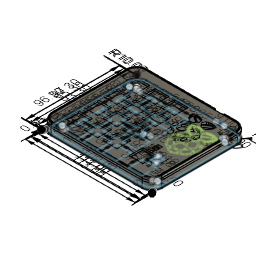
Raspberry pi pico Macropad (Autodesk Fusion 360 design; units mm, degrees)
Autodesk Fusion 360 part; units mm, degrees
sketch "Sketch1" plane through (0, 0, 0) normal (0, 0, 1) x (1, 0, 0)
  line L0 (12, 3) -> (101, 3)
  line L1 (111, 13) -> (111, 86.3)
  line L2 (101, 96.3) -> (12, 96.3)
  line L3 (2, 86.3) -> (2, 13)
  line L4 (11, 1) -> (102, 1)
  line L5 (112, 11) -> (112, 86.3)
  line L6 (102, 96.3) -> (11, 96.3)
  line L7 (1, 86.3) -> (1, 11)
  line L8 (10, 0) -> (103, 0)
  line L9 (113, 10) -> (113, 87.3)
  line L10 (103, 97.3) -> (10, 97.3)
  line L11 (0, 87.3) -> (0, 10)
  arc A0 (12, 96.3) -> (2, 86.3) centre (12, 86.3) ccw
  arc A1 (11, 96.3) -> (1, 86.3) centre (11, 86.3) ccw
  arc A2 (10, 97.3) -> (0, 87.3) centre (10, 87.3) ccw
  arc A3 (111, 86.3) -> (101, 96.3) centre (101, 86.3) ccw
  arc A4 (112, 86.3) -> (102, 96.3) centre (102, 86.3) ccw
  arc A5 (113, 87.3) -> (103, 97.3) centre (103, 87.3) ccw
  arc A6 (101, 3) -> (111, 13) centre (101, 13) ccw
  arc A7 (102, 1) -> (112, 11) centre (102, 11) ccw
  arc A8 (103, 0) -> (113, 10) centre (103, 10) ccw
  arc A9 (2, 13) -> (12, 3) centre (12, 13) ccw
  arc A10 (1, 11) -> (11, 1) centre (11, 11) ccw
  arc A11 (0, 10) -> (10, 0) centre (10, 10) ccw
  circle A12 centre (7, 82.9) radius 2.5
  circle A13 centre (105, 82.5) radius 2.5
  circle A14 centre (105, 13.8) radius 2.5
  circle A15 centre (7, 14.2) radius 2.5
  line L12 (56, 48.35) -> (56, 50.35)
  line L13 (56, 50.35) -> (53.5, 46.0199)
  line L14 (56, 50.35) -> (61, 50.35) construction
  line L15 (56, 50.35) -> (58.5, 46.0199)
  line L16 (58.5, 46.0199) -> (53.5, 46.0199)
  circle A16 centre (105, 13.8) radius 1.25
  circle A17 centre (105, 82.5) radius 1.25
  circle A18 centre (7, 82.9) radius 1.25
  circle A19 centre (7, 14.2) radius 1.25
  line L17 (0, 0) -> (0, 0.5)
  line L18 (0, 0.5) -> (0.5, 0.5)
  line L19 (10.5, 0.5) -> (102.5, 0.5)
  line L20 (112.5, 10.5) -> (112.5, 86.8)
  line L21 (102.5, 96.8) -> (10.5, 96.8)
  line L22 (0.5, 86.8) -> (0.5, 10.5)
  arc A20 (112.5, 86.8) -> (102.5, 96.8) centre (102.5, 86.8) ccw
  arc A21 (10.5, 96.8) -> (0.5, 86.8) centre (10.5, 86.8) ccw
  arc A22 (0.5, 10.5) -> (10.5, 0.5) centre (10.5, 10.5) ccw
  arc A23 (102.5, 0.5) -> (112.5, 10.5) centre (102.5, 10.5) ccw
  line L23 (90, 96.3) -> (81, 96.3)
  line L24 (81, 97.3) -> (90, 97.3)
  line L25 (81, 96.3) -> (90, 96.3)
  line L26 (91, 96.3) -> (82, 96.3)
  line L27 (91, 96.3) -> (82, 96.3)
  line L28 (82, 96.3) -> (82, 97.3)
  line L29 (82, 97.3) -> (91, 97.3)
  line L30 (91, 97.3) -> (91, 96.3)
  line L31 (90, 96.3) -> (81, 96.3)
  line L32 (81, 96.3) -> (81, 97.3)
  line L33 (81, 97.3) -> (90, 97.3)
  line L34 (90, 97.3) -> (90, 96.3)
  line L35 (16.9465, 83.797) -> (12.922, 83.797)
  line L36 (12.922, 83.797) -> (12.922, 84.0729)
  line L37 (12.922, 83.797) -> (26.9174, 83.797)
  line L38 (26.9174, 83.797) -> (26.9174, 69.8016)
  line L39 (26.9174, 69.8016) -> (12.922, 69.8016)
  line L40 (12.922, 69.8016) -> (12.922, 83.797)
  line L41 (26.9174, 83.797) -> (32.5054, 83.797)
  line L42 (32.5054, 83.797) -> (46.5008, 83.797)
  line L43 (46.5008, 83.797) -> (46.5008, 69.8016)
  line L44 (46.5008, 69.8016) -> (32.5054, 69.8016)
  line L45 (32.5054, 69.8016) -> (32.5054, 83.797)
  line L46 (46.5008, 83.797) -> (52.0888, 83.797)
  line L47 (52.0888, 83.797) -> (66.0842, 83.797)
  line L48 (66.0842, 83.797) -> (66.0842, 69.8016)
  line L49 (66.0842, 69.8016) -> (52.0888, 69.8016)
  line L50 (52.0888, 69.8016) -> (52.0888, 83.797)
  line L51 (12.922, 69.8016) -> (12.922, 64.2136)
  line L52 (12.922, 64.2136) -> (26.9174, 64.2136)
  line L53 (26.9174, 64.2136) -> (26.9174, 50.2182)
  line L54 (26.9174, 50.2182) -> (12.922, 50.2182)
  line L55 (12.922, 50.2182) -> (12.922, 64.2136)
  line L56 (26.9174, 64.2136) -> (32.5054, 64.2136)
  line L57 (32.5054, 64.2136) -> (46.5008, 64.2136)
  line L58 (46.5008, 64.2136) -> (46.5008, 50.2182)
  line L59 (46.5008, 50.2182) -> (32.5054, 50.2182)
  line L60 (32.5054, 50.2182) -> (32.5054, 64.2136)
  line L61 (46.5008, 64.2136) -> (52.0888, 64.2136)
  line L62 (52.0888, 64.2136) -> (66.0842, 64.2136)
  line L63 (66.0842, 64.2136) -> (66.0842, 50.2182)
  line L64 (66.0842, 50.2182) -> (52.0888, 50.2182)
  line L65 (52.0888, 50.2182) -> (52.0888, 64.2136)
  line L66 (12.922, 50.2182) -> (12.922, 44.6302)
  line L67 (12.922, 44.6302) -> (26.9174, 44.6302)
  line L68 (26.9174, 44.6302) -> (26.9174, 30.6348)
  line L69 (26.9174, 30.6348) -> (12.922, 30.6348)
  line L70 (12.922, 30.6348) -> (12.922, 44.6302)
  line L71 (32.5054, 44.6302) -> (46.5008, 44.6302)
  line L72 (46.5008, 44.6302) -> (46.5008, 30.6348)
  line L73 (46.5008, 30.6348) -> (32.5054, 30.6348)
  line L74 (32.5054, 30.6348) -> (32.5054, 44.6302)
  line L75 (52.0888, 44.6302) -> (66.0842, 44.6302)
  line L76 (66.0842, 44.6302) -> (66.0842, 30.6348)
  line L77 (66.0842, 30.6348) -> (52.0888, 30.6348)
  line L78 (52.0888, 30.6348) -> (52.0888, 44.6302)
  line L79 (12.922, 30.6348) -> (12.922, 25.0468)
  line L80 (12.922, 25.0468) -> (26.9174, 25.0468)
  line L81 (26.9174, 25.0468) -> (26.9174, 11.0514)
  line L82 (26.9174, 11.0514) -> (12.922, 11.0514)
  line L83 (12.922, 11.0514) -> (12.922, 25.0468)
  line L84 (32.5054, 25.0468) -> (46.5008, 25.0468)
  line L85 (46.5008, 25.0468) -> (46.5008, 11.0514)
  line L86 (46.5008, 11.0514) -> (32.5054, 11.0514)
  line L87 (32.5054, 11.0514) -> (32.5054, 25.0468)
  line L88 (52.0888, 25.0468) -> (66.0842, 25.0468)
  line L89 (66.0842, 25.0468) -> (66.0842, 11.0514)
  line L90 (66.0842, 11.0514) -> (52.0888, 11.0514)
  line L91 (52.0888, 11.0514) -> (52.0888, 25.0468)
  line L92 (78.4702, 25.0468) -> (92.4656, 25.0468)
  line L93 (92.4656, 25.0468) -> (92.4656, 11.0514)
  line L94 (92.4656, 11.0514) -> (78.4702, 11.0514)
  line L95 (78.4702, 11.0514) -> (78.4702, 25.0468)
  line L96 (83.3562, 29.7458) -> (87.6742, 29.7458)
  line L97 (87.6742, 29.7458) -> (87.6742, 32.2858)
  line L98 (87.6742, 32.2858) -> (83.3562, 32.2858)
  line L99 (83.3562, 32.2858) -> (83.3562, 29.7458)
  line L100 (83.3562, 32.2858) -> (83.3562, 33.3018)
  line L101 (83.3562, 33.3018) -> (87.6742, 33.3018)
  line L102 (87.6742, 33.3018) -> (87.6742, 35.8418)
  line L103 (87.6742, 35.8418) -> (83.3562, 35.8418)
  line L104 (83.3562, 35.8418) -> (83.3562, 33.3018)
  spline S0 degree 3 poles (79.019, 82.9251) (78.832, 82.9193) (78.6306, 82.8502) (78.4021, 82.67) knots 0 0 0 0 1 1 1 1
  spline S1 degree 3 poles (78.4021, 82.67) (77.8427, 82.8857) (77.2999, 82.9607) (76.8147, 82.5215) knots 0 0 0 0 1 1 1 1
  spline S2 degree 3 poles (76.8147, 82.5215) (76.0654, 82.6186) (75.822, 82.4181) (75.6375, 82.1839) knots 0 0 0 0 1 1 1 1
  spline S3 degree 3 poles (75.6375, 82.1839) (75.473, 82.1873) (74.4067, 82.353) (73.9177, 81.6236) knots 0 0 0 0 1 1 1 1
  spline S4 degree 3 poles (73.9177, 81.6236) (72.6889, 81.7689) (72.3005, 80.9008) (72.7406, 80.0911) knots 0 0 0 0 1 1 1 1
  spline S5 degree 3 poles (72.7406, 80.0911) (72.4896, 79.7027) (72.2295, 79.3188) (72.8164, 78.5781) knots 0 0 0 0 1 1 1 1
  spline S6 degree 3 poles (72.8164, 78.5781) (72.6088, 78.1656) (72.7375, 77.7181) (73.2266, 77.1765) knots 0 0 0 0 1 1 1 1
  spline S7 degree 3 poles (73.2266, 77.1765) (73.0976, 76.5965) (73.3513, 76.1874) (73.8064, 75.8685) knots 0 0 0 0 1 1 1 1
  spline S8 degree 3 poles (73.8064, 75.8685) (73.7212, 75.0749) (74.5341, 74.6135) (74.7768, 74.4491) knots 0 0 0 0 1 1 1 1
  spline S9 degree 3 poles (74.7768, 74.4491) (74.87, 73.9867) (75.0642, 73.5503) (75.9927, 73.3091) knots 0 0 0 0 1 1 1 1
  spline S10 degree 3 poles (75.9927, 73.3091) (76.1459, 72.6199) (76.7038, 72.5009) (77.2442, 72.3563) knots 0 0 0 0 1 1 1 1
  spline S11 degree 3 poles (77.2442, 72.3563) (75.4583, 71.3182) (73.9267, 69.9524) (73.9371, 66.601) knots 0 0 0 0 1 1 1 1
  line L105 (73.9371, 66.601) -> (73.6755, 66.1343)
  spline S12 degree 3 poles (73.6755, 66.1343) (71.6276, 64.889) (69.7852, 60.8863) (72.6664, 57.633) knots 0 0 0 0 1 1 1 1
  spline S13 degree 3 poles (72.6664, 57.633) (72.8545, 56.6146) (73.1701, 55.8831) (73.4511, 55.0736) knots 0 0 0 0 1 1 1 1
  spline S14 degree 3 poles (73.4511, 55.0736) (73.8714, 51.8114) (76.6144, 50.2838) (77.338, 50.1032) knots 0 0 0 0 1 1 1 1
  spline S15 degree 3 poles (77.338, 50.1032) (78.3981, 49.2956) (79.5273, 48.5294) (81.0554, 47.9926) knots 0 0 0 0 1 1 1 1
  spline S16 degree 3 poles (81.0554, 47.9926) (82.4956, 46.5072) (84.0561, 45.9409) (85.6251, 45.9419) knots 0 0 0 0 1 1 1 1
  spline S17 degree 3 poles (85.6251, 45.9419) (85.6482, 45.9419) (88.824, 46.507) (90.2645, 47.9926) knots 0 0 0 0 1 1 1 1
  spline S18 degree 3 poles (90.2645, 47.9926) (91.7924, 48.5294) (92.9215, 49.2956) (93.9818, 50.1032) knots 0 0 0 0 1 1 1 1
  spline S19 degree 3 poles (93.9818, 50.1032) (94.7052, 50.2838) (97.4482, 51.8114) (97.8685, 55.0736) knots 0 0 0 0 1 1 1 1
  spline S20 degree 3 poles (97.8685, 55.0736) (98.1495, 55.8831) (98.4651, 56.6146) (98.6534, 57.633) knots 0 0 0 0 1 1 1 1
  spline S21 degree 3 poles (98.6534, 57.633) (101.5343, 60.8866) (99.692, 64.8894) (97.6443, 66.1348) knots 0 0 0 0 1 1 1 1
  line L106 (97.6443, 66.1348) -> (97.3821, 66.6014)
  spline S22 degree 3 poles (97.3821, 66.6014) (97.3925, 69.9525) (95.861, 71.3184) (94.0751, 72.3568) knots 0 0 0 0 1 1 1 1
  spline S23 degree 3 poles (94.0751, 72.3568) (94.6154, 72.5014) (95.1735, 72.6204) (95.3265, 73.3096) knots 0 0 0 0 1 1 1 1
  spline S24 degree 3 poles (95.3265, 73.3096) (96.2549, 73.5509) (96.4493, 73.9872) (96.5424, 74.4496) knots 0 0 0 0 1 1 1 1
  spline S25 degree 3 poles (96.5424, 74.4496) (96.7852, 74.6139) (97.598, 75.0754) (97.513, 75.869) knots 0 0 0 0 1 1 1 1
  spline S26 degree 3 poles (97.513, 75.869) (97.9679, 76.1879) (98.2217, 76.5971) (98.0926, 77.177) knots 0 0 0 0 1 1 1 1
  spline S27 degree 3 poles (98.0926, 77.177) (98.5818, 77.7185) (98.7104, 78.166) (98.5028, 78.5786) knots 0 0 0 0 1 1 1 1
  spline S28 degree 3 poles (98.5028, 78.5786) (99.0899, 79.3189) (98.8294, 79.7028) (98.5787, 80.0913) knots 0 0 0 0 1 1 1 1
  spline S29 degree 3 poles (98.5787, 80.0913) (99.0185, 80.9009) (98.6304, 81.7692) (97.4011, 81.6237) knots 0 0 0 0 1 1 1 1
  spline S30 degree 3 poles (97.4011, 81.6237) (96.9124, 82.3531) (95.8463, 82.1875) (95.6814, 82.1841) knots 0 0 0 0 1 1 1 1
  spline S31 degree 3 poles (95.6814, 82.1841) (95.497, 82.4182) (95.2535, 82.6188) (94.5043, 82.5216) knots 0 0 0 0 1 1 1 1
  spline S32 degree 3 poles (94.5043, 82.5216) (94.0191, 82.9609) (93.4765, 82.886) (92.9169, 82.6701) knots 0 0 0 0 1 1 1 1
  spline S33 degree 3 poles (92.9169, 82.6701) (92.2524, 83.1945) (91.8127, 82.7742) (91.3104, 82.6153) knots 0 0 0 0 1 1 1 1
  spline S34 degree 3 poles (91.3104, 82.6153) (90.5059, 82.8782) (90.3218, 82.5181) (89.9266, 82.3714) knots 0 0 0 0 1 1 1 1
  spline S35 degree 3 poles (89.9266, 82.3714) (89.0491, 82.5568) (88.7825, 82.1531) (88.362, 81.7271) knots 0 0 0 0 1 1 1 1
  line L107 (88.362, 81.7271) -> (87.8726, 81.7368)
  spline S36 degree 3 poles (87.8726, 81.7368) (86.5492, 80.9569) (85.8917, 79.3688) (85.6587, 78.5524) knots 0 0 0 0 1 1 1 1
  spline S37 degree 3 poles (85.6587, 78.5524) (85.4256, 79.3689) (84.7696, 80.957) (83.4465, 81.7368) knots 0 0 0 0 1 1 1 1
  line L108 (83.4465, 81.7368) -> (82.9572, 81.7271)
  spline S38 degree 3 poles (82.9572, 81.7271) (82.536, 82.1531) (82.2695, 82.5568) (81.3921, 82.3713) knots 0 0 0 0 1 1 1 1
  spline S39 degree 3 poles (81.3921, 82.3713) (80.9967, 82.5181) (80.8134, 82.8782) (80.0082, 82.6153) knots 0 0 0 0 1 1 1 1
  spline S40 degree 3 poles (80.0082, 82.6153) (79.6785, 82.7196) (79.3753, 82.9363) (79.0184, 82.9252) knots 0 0 0 0 1 1 1 1
  spline S41 degree 3 poles (76.3842, 79.494) (79.8953, 77.6839) (81.9364, 76.2196) (83.0547, 74.9724) knots 0 0 0 0 1 1 1 1
  spline S42 degree 3 poles (83.0547, 74.9724) (82.482, 72.6772) (79.4946, 72.5724) (78.4022, 72.6368) knots 0 0 0 0 1 1 1 1
  spline S43 degree 3 poles (78.4022, 72.6368) (78.6258, 72.7409) (78.8125, 72.8657) (78.8787, 73.0572) knots 0 0 0 0 1 1 1 1
  spline S44 degree 3 poles (78.8787, 73.0572) (78.6046, 73.252) (77.6327, 73.0778) (76.9542, 73.4589) knots 0 0 0 0 1 1 1 1
  spline S45 degree 3 poles (76.9542, 73.4589) (77.2148, 73.513) (77.3368, 73.5656) (77.4586, 73.7579) knots 0 0 0 0 1 1 1 1
  spline S46 degree 3 poles (77.4586, 73.7579) (76.8176, 73.9623) (76.1271, 74.1386) (75.7209, 74.4773) knots 0 0 0 0 1 1 1 1
  spline S47 degree 3 poles (75.7209, 74.4773) (75.9401, 74.4746) (76.1447, 74.4282) (76.4309, 74.6267) knots 0 0 0 0 1 1 1 1
  spline S48 degree 3 poles (76.4309, 74.6267) (75.8568, 74.9361) (75.2441, 75.1814) (74.7681, 75.6544) knots 0 0 0 0 1 1 1 1
  spline S49 degree 3 poles (74.7681, 75.6544) (75.0649, 75.6616) (75.385, 75.6573) (75.4781, 75.7665) knots 0 0 0 0 1 1 1 1
  spline S50 degree 3 poles (75.4781, 75.7665) (74.9526, 76.0921) (74.5091, 76.4541) (74.1421, 76.8501) knots 0 0 0 0 1 1 1 1
  spline S51 degree 3 poles (74.1421, 76.8501) (74.5575, 76.8) (74.733, 76.8431) (74.8335, 76.9155) knots 0 0 0 0 1 1 1 1
  spline S52 degree 3 poles (74.8335, 76.9155) (74.4361, 77.3224) (73.9334, 77.666) (73.6937, 78.1674) knots 0 0 0 0 1 1 1 1
  spline S53 degree 3 poles (73.6937, 78.1674) (74.0021, 78.0611) (74.2843, 78.0203) (74.4877, 78.1767) knots 0 0 0 0 1 1 1 1
  spline S54 degree 3 poles (74.4877, 78.1767) (74.3528, 78.4812) (73.7745, 78.6609) (73.4414, 79.3725) knots 0 0 0 0 1 1 1 1
  spline S55 degree 3 poles (73.4414, 79.3725) (73.7662, 79.341) (74.1106, 79.3017) (74.1795, 79.3725) knots 0 0 0 0 1 1 1 1
  spline S56 degree 3 poles (74.1795, 79.3725) (74.0288, 79.9866) (73.7702, 80.3319) (73.5165, 80.6896) knots 0 0 0 0 1 1 1 1
  spline S57 degree 3 poles (73.5165, 80.6896) (74.2115, 80.6999) (75.2645, 80.6869) (75.2168, 80.7456) knots 0 0 0 0 1 1 1 1
  line L109 (75.2168, 80.7456) -> (74.7871, 81.1846)
  spline S58 degree 3 poles (74.7871, 81.1846) (75.466, 81.3675) (76.1606, 81.1553) (76.6649, 80.9979) knots 0 0 0 0 1 1 1 1
  spline S59 degree 3 poles (76.6649, 80.9979) (76.8913, 81.1765) (76.6608, 81.4024) (76.3846, 81.6331) knots 0 0 0 0 1 1 1 1
  spline S60 degree 3 poles (76.3846, 81.6331) (76.9615, 81.556) (77.4828, 81.4234) (77.9541, 81.2407) knots 0 0 0 0 1 1 1 1
  spline S61 degree 3 poles (77.9541, 81.2407) (78.2058, 81.468) (77.7906, 81.6954) (77.5897, 81.9227) knots 0 0 0 0 1 1 1 1
  spline S62 degree 3 poles (77.5897, 81.9227) (78.481, 81.7537) (78.8587, 81.516) (79.2339, 81.2781) knots 0 0 0 0 1 1 1 1
  spline S63 degree 3 poles (79.2339, 81.2781) (79.5062, 81.5391) (79.2495, 81.7609) (79.0658, 81.9881) knots 0 0 0 0 1 1 1 1
  spline S64 degree 3 poles (79.0658, 81.9881) (79.7379, 81.7392) (80.0841, 81.4178) (80.4485, 81.1006) knots 0 0 0 0 1 1 1 1
  spline S65 degree 3 poles (80.4485, 81.1006) (80.572, 81.2673) (80.7624, 81.3896) (80.5325, 81.7919) knots 0 0 0 0 1 1 1 1
  spline S66 degree 3 poles (80.5325, 81.7919) (81.0097, 81.5169) (81.3691, 81.1928) (81.6349, 80.8296) knots 0 0 0 0 1 1 1 1
  spline S67 degree 3 poles (81.6349, 80.8296) (81.9302, 81.0177) (81.8109, 81.2747) (81.8124, 81.5117) knots 0 0 0 0 1 1 1 1
  spline S68 degree 3 poles (81.8124, 81.5117) (82.3084, 81.1083) (82.6231, 80.679) (83.0083, 80.2598) knots 0 0 0 0 1 1 1 1
  spline S69 degree 3 poles (83.0083, 80.2598) (83.0859, 80.3164) (83.1538, 80.5079) (83.2139, 80.811) knots 0 0 0 0 1 1 1 1
  spline S70 degree 3 poles (83.2139, 80.811) (84.3968, 79.6633) (86.0685, 76.7723) (83.6435, 75.6261) knots 0 0 0 0 1 1 1 1
  spline S71 degree 3 poles (83.6435, 75.6261) (81.5797, 77.3282) (79.1149, 78.5655) (76.3834, 79.4936) knots 0 0 0 0 1 1 1 1
  line L110 (76.3834, 79.4936) -> (76.3842, 79.494)
  spline S72 degree 3 poles (95.0139, 79.494) (91.5033, 77.6837) (89.4622, 76.2198) (88.344, 74.9724) knots 0 0 0 0 1 1 1 1
  spline S73 degree 3 poles (88.344, 74.9724) (88.9167, 72.6772) (91.904, 72.5724) (92.9964, 72.6368) knots 0 0 0 0 1 1 1 1
  spline S74 degree 3 poles (92.9964, 72.6368) (92.7727, 72.7409) (92.5861, 72.8657) (92.52, 73.0572) knots 0 0 0 0 1 1 1 1
  spline S75 degree 3 poles (92.52, 73.0572) (92.7941, 73.252) (93.766, 73.0778) (94.4444, 73.4589) knots 0 0 0 0 1 1 1 1
  spline S76 degree 3 poles (94.4444, 73.4589) (94.1838, 73.513) (94.0619, 73.5656) (93.94, 73.7579) knots 0 0 0 0 1 1 1 1
  spline S77 degree 3 poles (93.94, 73.7579) (94.5811, 73.9623) (95.2716, 74.1386) (95.6776, 74.4773) knots 0 0 0 0 1 1 1 1
  spline S78 degree 3 poles (95.6776, 74.4773) (95.4585, 74.4746) (95.2539, 74.4282) (94.9676, 74.6267) knots 0 0 0 0 1 1 1 1
  spline S79 degree 3 poles (94.9676, 74.6267) (95.5419, 74.9361) (96.1546, 75.1814) (96.6306, 75.6544) knots 0 0 0 0 1 1 1 1
  spline S80 degree 3 poles (96.6306, 75.6544) (96.3337, 75.6616) (96.0136, 75.6573) (95.9206, 75.7665) knots 0 0 0 0 1 1 1 1
  spline S81 degree 3 poles (95.9206, 75.7665) (96.4461, 76.0921) (96.8896, 76.4541) (97.2566, 76.8501) knots 0 0 0 0 1 1 1 1
  spline S82 degree 3 poles (97.2566, 76.8501) (96.841, 76.8) (96.6657, 76.8431) (96.5652, 76.9155) knots 0 0 0 0 1 1 1 1
  spline S83 degree 3 poles (96.5652, 76.9155) (96.9624, 77.3224) (97.4653, 77.666) (97.705, 78.1674) knots 0 0 0 0 1 1 1 1
  spline S84 degree 3 poles (97.705, 78.1674) (97.3965, 78.0611) (97.1143, 78.0203) (96.9108, 78.1767) knots 0 0 0 0 1 1 1 1
  spline S85 degree 3 poles (96.9108, 78.1767) (97.0458, 78.4812) (97.6242, 78.6609) (97.9572, 79.3725) knots 0 0 0 0 1 1 1 1
  spline S86 degree 3 poles (97.9572, 79.3725) (97.6325, 79.341) (97.288, 79.3017) (97.2191, 79.3725) knots 0 0 0 0 1 1 1 1
  spline S87 degree 3 poles (97.2191, 79.3725) (97.3701, 79.9868) (97.6288, 80.3321) (97.8824, 80.6898) knots 0 0 0 0 1 1 1 1
  spline S88 degree 3 poles (97.8824, 80.6898) (97.1874, 80.7001) (96.1345, 80.6871) (96.1821, 80.7458) knots 0 0 0 0 1 1 1 1
  line L111 (96.1821, 80.7458) -> (96.6119, 81.185)
  spline S89 degree 3 poles (96.6119, 81.185) (95.933, 81.3677) (95.2384, 81.1556) (94.734, 80.9981) knots 0 0 0 0 1 1 1 1
  spline S90 degree 3 poles (94.734, 80.9981) (94.5077, 81.1767) (94.738, 81.4026) (95.0143, 81.6333) knots 0 0 0 0 1 1 1 1
  spline S91 degree 3 poles (95.0143, 81.6333) (94.4374, 81.5564) (93.916, 81.4237) (93.4448, 81.241) knots 0 0 0 0 1 1 1 1
  spline S92 degree 3 poles (93.4448, 81.241) (93.193, 81.4682) (93.6083, 81.6956) (93.8092, 81.9229) knots 0 0 0 0 1 1 1 1
  spline S93 degree 3 poles (93.8092, 81.9229) (92.9179, 81.7539) (92.5403, 81.5162) (92.1649, 81.2783) knots 0 0 0 0 1 1 1 1
  spline S94 degree 3 poles (92.1649, 81.2783) (91.8926, 81.5393) (92.1494, 81.7611) (92.3331, 81.9883) knots 0 0 0 0 1 1 1 1
  spline S95 degree 3 poles (92.3331, 81.9883) (91.661, 81.7394) (91.3149, 81.418) (90.9505, 81.1008) knots 0 0 0 0 1 1 1 1
  spline S96 degree 3 poles (90.9505, 81.1008) (90.8268, 81.2676) (90.6365, 81.3898) (90.8663, 81.7921) knots 0 0 0 0 1 1 1 1
  spline S97 degree 3 poles (90.8663, 81.7921) (90.3892, 81.5171) (90.0298, 81.193) (89.764, 80.8299) knots 0 0 0 0 1 1 1 1
  spline S98 degree 3 poles (89.764, 80.8299) (89.4687, 81.0179) (89.5881, 81.275) (89.5865, 81.5119) knots 0 0 0 0 1 1 1 1
  spline S99 degree 3 poles (89.5865, 81.5119) (89.0905, 81.1085) (88.7758, 80.6793) (88.3906, 80.26) knots 0 0 0 0 1 1 1 1
  spline S100 degree 3 poles (88.3906, 80.26) (88.313, 80.3166) (88.2451, 80.5081) (88.1851, 80.8113) knots 0 0 0 0 1 1 1 1
  spline S101 degree 3 poles (88.1851, 80.8113) (87.0021, 79.6635) (85.3304, 76.7725) (87.7554, 75.6263) knots 0 0 0 0 1 1 1 1
  spline S102 degree 3 poles (87.7554, 75.6263) (89.8181, 77.3289) (92.2828, 78.5659) (95.0144, 79.494) knots 0 0 0 0 1 1 1 1
  line L112 (95.0144, 79.494) -> (95.0139, 79.494)
  spline S103 degree 3 poles (89.9511, 56.1219) (89.9633, 53.9801) (88.0903, 52.2346) (85.7676, 52.2234) knots 0 0 0 0 1 1 1 1
  spline S104 degree 3 poles (85.7676, 52.2234) (83.4449, 52.2121) (81.552, 53.9392) (81.5398, 56.0811) knots 0 0 0 0 1 1 1 1
  arc A24 (81.5398, 56.0811) -> (81.5398, 56.1219) centre (83.9969, 56.1015) cw
  spline S105 degree 3 poles (81.5398, 56.1219) (81.5276, 58.2636) (83.4005, 60.0091) (85.7233, 60.0204) knots 0 0 0 0 1 1 1 1
  spline S106 degree 3 poles (85.7233, 60.0204) (88.046, 60.0317) (89.9388, 58.3046) (89.9511, 56.1627) knots 0 0 0 0 1 1 1 1
  line L113 (89.9511, 56.1627) -> (89.9511, 56.1219)
  spline S107 degree 3 poles (83.312, 67.2004) (85.0546, 66.0586) (85.3687, 63.4707) (84.0136, 61.4201) knots 0 0 0 0 1 1 1 1
  spline S108 degree 3 poles (84.0136, 61.4201) (82.6584, 59.3695) (80.1472, 58.6326) (78.4046, 59.7742) knots 0 0 0 0 1 1 1 1
  spline S109 degree 3 poles (78.4046, 59.7742) (76.6619, 60.916) (76.3479, 63.504) (77.7029, 65.5545) knots 0 0 0 0 1 1 1 1
  spline S110 degree 3 poles (77.7029, 65.5545) (79.0581, 67.6052) (81.5693, 68.3421) (83.312, 67.2004) knots 0 0 0 0 1 1 1 1
  spline S111 degree 3 poles (88.0154, 67.4071) (86.2729, 66.2654) (85.9587, 63.6774) (87.3137, 61.6268) knots 0 0 0 0 1 1 1 1
  spline S112 degree 3 poles (87.3137, 61.6268) (88.6689, 59.5762) (91.1801, 58.8392) (92.9227, 59.981) knots 0 0 0 0 1 1 1 1
  spline S113 degree 3 poles (92.9227, 59.981) (94.6654, 61.1227) (94.9795, 63.7106) (93.6244, 65.7613) knots 0 0 0 0 1 1 1 1
  spline S114 degree 3 poles (93.6244, 65.7613) (92.2693, 67.8119) (89.7581, 68.5488) (88.0154, 67.4071) knots 0 0 0 0 1 1 1 1
  spline S115 degree 3 poles (74.6024, 65.3338) (76.4839, 65.8381) (75.2377, 57.5503) (73.7068, 58.2303) knots 0 0 0 0 1 1 1 1
  spline S116 degree 3 poles (73.7068, 58.2303) (72.0229, 59.5846) (71.4806, 63.551) (74.6024, 65.3338) knots 0 0 0 0 1 1 1 1
  spline S117 degree 3 poles (96.3451, 65.4371) (94.4634, 65.9413) (95.7099, 57.6531) (97.2407, 58.3331) knots 0 0 0 0 1 1 1 1
  spline S118 degree 3 poles (97.2407, 58.3331) (98.9246, 59.6876) (99.467, 63.6544) (96.3451, 65.4371) knots 0 0 0 0 1 1 1 1
  spline S119 degree 3 poles (89.9526, 71.609) (93.1995, 72.1572) (95.9012, 70.2282) (95.7921, 66.7074) knots 0 0 0 0 1 1 1 1
  spline S120 degree 3 poles (95.7921, 66.7074) (95.6853, 65.3576) (88.7564, 71.408) (89.9526, 71.609) knots 0 0 0 0 1 1 1 1
  spline S121 degree 3 poles (80.9815, 71.7123) (77.7344, 72.2606) (75.0329, 70.3311) (75.142, 66.8106) knots 0 0 0 0 1 1 1 1
  spline S122 degree 3 poles (75.142, 66.8106) (75.2487, 65.4609) (82.1778, 71.5113) (80.9815, 71.7123) knots 0 0 0 0 1 1 1 1
  spline S123 degree 3 poles (85.6456, 72.5334) (83.7077, 72.5838) (81.8478, 71.0952) (81.8433, 70.2317) knots 0 0 0 0 1 1 1 1
  spline S124 degree 3 poles (81.8433, 70.2317) (81.838, 69.1825) (83.3755, 68.1083) (85.6588, 68.081) knots 0 0 0 0 1 1 1 1
  spline S125 degree 3 poles (85.6588, 68.081) (87.9904, 68.0644) (89.4782, 68.9409) (89.4857, 70.0236) knots 0 0 0 0 1 1 1 1
  spline S126 degree 3 poles (89.4857, 70.0236) (89.4943, 71.2504) (87.3651, 72.5524) (85.6456, 72.5335) knots 0 0 0 0 1 1 1 1
  line L114 (85.6456, 72.5335) -> (85.6456, 72.5334)
  spline S127 degree 3 poles (85.7639, 51.0187) (87.4535, 51.0925) (89.7205, 50.4746) (89.7251, 49.6547) knots 0 0 0 0 1 1 1 1
  spline S128 degree 3 poles (89.7251, 49.6547) (89.7531, 48.8587) (87.669, 47.0602) (85.6519, 47.095) knots 0 0 0 0 1 1 1 1
  spline S129 degree 3 poles (85.6519, 47.095) (83.5629, 47.0048) (81.5145, 48.8061) (81.5413, 49.4305) knots 0 0 0 0 1 1 1 1
  spline S130 degree 3 poles (81.5413, 49.4305) (81.5099, 50.3459) (84.0848, 51.0607) (85.7639, 51.0187) knots 0 0 0 0 1 1 1 1
  spline S131 degree 3 poles (79.5233, 55.877) (80.7262, 54.4278) (81.2746, 51.8818) (80.2707, 51.1311) knots 0 0 0 0 1 1 1 1
  spline S132 degree 3 poles (80.2707, 51.1311) (79.321, 50.5582) (77.0147, 50.7941) (75.3755, 53.1491) knots 0 0 0 0 1 1 1 1
  spline S133 degree 3 poles (75.3755, 53.1491) (74.2699, 55.1252) (74.4123, 57.1361) (75.1886, 57.7269) knots 0 0 0 0 1 1 1 1
  spline S134 degree 3 poles (75.1886, 57.7269) (76.3494, 58.4339) (78.1429, 57.4788) (79.5234, 55.877) knots 0 0 0 0 1 1 1 1
  line L115 (79.5234, 55.877) -> (79.5233, 55.877)
  spline S135 degree 3 poles (91.7637, 56.3364) (90.4622, 54.812) (89.7375, 52.0315) (90.6869, 51.136) knots 0 0 0 0 1 1 1 1
  spline S136 degree 3 poles (90.6869, 51.136) (91.5947, 50.4403) (94.0317, 50.5376) (95.8318, 53.0353) knots 0 0 0 0 1 1 1 1
  spline S137 degree 3 poles (95.8318, 53.0353) (97.1389, 54.7129) (96.701, 57.5145) (95.9543, 58.2584) knots 0 0 0 0 1 1 1 1
  spline S138 degree 3 poles (95.9543, 58.2584) (94.8452, 59.1163) (93.253, 58.0184) (91.7637, 56.3368) knots 0 0 0 0 1 1 1 1
  line L116 (91.7637, 56.3368) -> (91.7637, 56.3364)
  circle A25 centre (100.0119, 84.9707) radius 2
  line L117 (82.3562, 35.8418) -> (82.3562, 36.8418)
  line L118 (82.3562, 36.8418) -> (83.3562, 36.8418)
  line L119 (88.6742, 29.7458) -> (88.6742, 28.7458)
  line L120 (88.6742, 28.7458) -> (87.6742, 28.7458)
  line L121 (88.6742, 28.7458) -> (82.3562, 28.7458)
  line L122 (82.3562, 28.7458) -> (82.3562, 36.8418)
  line L123 (82.3562, 36.8418) -> (88.6742, 36.8418)
  line L124 (88.6742, 36.8418) -> (88.6742, 28.7458)
  point P0 (2, 3)
  point P1 (111, 3)
  point P2 (2, 96.3)
  point P3 (1, 1)
  point P4 (112, 1)
  point P5 (1, 96.3)
  point P6 (113, 0)
  point P7 (0, 97.3)
  point P8 (112.5, 0.5)
  point P9 (0.5, 96.8)
  dimension "d3" = 109
  dimension "d4" = 93.3
  dimension "d7" = 111
  dimension "d8" = 95.3
  dimension "d9" = 113
  dimension "d10" = 97.3
  dimension "d11" = 10
  dimension "d14" = 5
  dimension "d18" = 5
  dimension "d21" = 5
  dimension "d24" = 5
  dimension "d32" = 2
  dimension "d33" = 120
  dimension "d34" = 5
  dimension "d35" = 5
  dimension "d38" = 2.5
  dimension "d39" = 2.5
  dimension "d40" = 2.5
  dimension "d41" = 2.5
  dimension "d42" = 0.5
  dimension "d43" = 0.5
  dimension "d44" = 112
  dimension "d45" = 96.3
  dimension "d46" = 10
  dimension "d47" = 10
  dimension "d64" = 9
  dimension "d107" = 13.9954
  dimension "d108" = 13.9954
  dimension "d109" = 5.588
  dimension "d110" = 13.9954
  dimension "d111" = 13.9954
  dimension "d112" = 5.588
  dimension "d113" = 13.9954
  dimension "d114" = 13.9954
  dimension "d115" = 5.588
  dimension "d116" = 13.9954
  dimension "d117" = 13.9954
  dimension "d118" = 5.588
  dimension "d119" = 13.9954
  dimension "d120" = 13.9954
  dimension "d121" = 5.588
  dimension "d122" = 13.9954
  dimension "d123" = 13.9954
  dimension "d124" = 5.588
  dimension "d125" = 13.9954
  dimension "d126" = 13.9954
  dimension "d127" = 13.9954
  dimension "d128" = 13.9954
  dimension "d129" = 13.9954
  dimension "d130" = 13.9954
  dimension "d131" = 5.588
  dimension "d132" = 13.9954
  dimension "d133" = 13.9954
  dimension "d134" = 13.9954
  dimension "d135" = 13.9954
  dimension "d136" = 13.9954
  dimension "d137" = 13.9954
  dimension "d139" = 13.9954
  dimension "d140" = 13.9954
  dimension "d143" = 4.318
  dimension "d144" = 2.54
  dimension "d145" = 1.016
  dimension "d146" = 4.318
  dimension "d147" = 2.54
  dimension "d175" = 4
  dimension "d186" = 1
  constraint horizontal L0
  constraint vertical L1
  constraint horizontal L2
  constraint vertical L3
  constraint horizontal L4
  constraint vertical L5
  constraint horizontal L6
  constraint vertical L7
  constraint horizontal L8
  constraint vertical L9
  constraint horizontal L10
  constraint vertical L11
  constraint coincident L17.start origin
  constraint coincident P2 L2
  constraint coincident P2 L3
  constraint tangent L2 A0
  constraint tangent L3 A0
  constraint coincident P5 L6
  constraint coincident P5 L7
  constraint tangent L6 A1
  constraint tangent L7 A1
  constraint equal A0 A1
  constraint coincident P7 L10
  constraint coincident P7 L11
  constraint tangent L10 A2
  constraint tangent L11 A2
  constraint equal A0 A2
  constraint tangent L1 A3
  constraint tangent L2 A3
  constraint equal A0 A3
  constraint tangent L5 A4
  constraint tangent L6 A4
  constraint equal A0 A4
  constraint tangent L9 A5
  constraint tangent L10 A5
  constraint equal A0 A5
  constraint coincident P1 L0
  constraint coincident P1 L1
  constraint tangent L0 A6
  constraint tangent L1 A6
  constraint equal A0 A6
  constraint coincident P4 L4
  constraint coincident P4 L5
  constraint tangent L4 A7
  constraint tangent L5 A7
  constraint equal A0 A7
  constraint coincident P6 L8
  constraint coincident P6 L9
  constraint tangent L8 A8
  constraint tangent L9 A8
  constraint equal A0 A8
  constraint coincident P0 L0
  constraint coincident P0 L3
  constraint tangent L0 A9
  constraint tangent L3 A9
  constraint equal A0 A9
  constraint coincident P3 L4
  constraint coincident P3 L7
  constraint tangent L4 A10
  constraint tangent L7 A10
  constraint equal A0 A10
  constraint coincident L17.start L8
  constraint coincident L17.start L11
  constraint tangent L8 A11
  constraint tangent L11 A11
  constraint equal A0 A11
  constraint vertical L12
  constraint horizontal L14
  constraint horizontal L16
  constraint concentric A14 A16
  constraint concentric A13 A17
  constraint concentric A12 A18
  constraint concentric A15 A19
  constraint vertical L17
  constraint perpendicular L17 L18
  constraint horizontal L19
  constraint vertical L20
  constraint horizontal L21
  constraint vertical L22
  constraint tangent L20 A20
  constraint tangent L21 A20
  constraint coincident P9 L21
  constraint coincident P9 L22
  constraint tangent L21 A21
  constraint tangent L22 A21
  constraint coincident L18.end L19
  constraint coincident L18.end L22
  constraint tangent L19 A22
  constraint tangent L22 A22
  constraint equal A21 A22
  constraint coincident P8 L19
  constraint coincident P8 L20
  constraint tangent L19 A23
  constraint tangent L20 A23
  constraint equal A21 A23
  constraint coincident L2 L23.start
  constraint horizontal L23
  constraint horizontal L24
  constraint horizontal L25
  constraint coincident L2 L26.start
  constraint horizontal L26
  constraint horizontal L27
  constraint vertical L28
  constraint horizontal L29
  constraint vertical L30
  constraint horizontal L31
  constraint vertical L32
  constraint horizontal L33
  constraint vertical L34
  constraint horizontal L35
  constraint vertical L36
  constraint horizontal L37
  constraint vertical L38
  constraint horizontal L39
  constraint vertical L40
  constraint perpendicular L38 L41
  constraint horizontal L42
  constraint vertical L43
  constraint horizontal L44
  constraint vertical L45
  constraint perpendicular L43 L46
  constraint horizontal L47
  constraint vertical L48
  constraint horizontal L49
  constraint vertical L50
  constraint perpendicular L39 L51
  constraint horizontal L52
  constraint vertical L53
  constraint horizontal L54
  constraint vertical L55
  constraint perpendicular L53 L56
  constraint horizontal L57
  constraint vertical L58
  constraint horizontal L59
  constraint vertical L60
  constraint perpendicular L58 L61
  constraint horizontal L62
  constraint vertical L63
  constraint horizontal L64
  constraint vertical L65
  constraint perpendicular L54 L66
  constraint horizontal L67
  constraint vertical L68
  constraint horizontal L69
  constraint vertical L70
  constraint horizontal L71
  constraint vertical L72
  constraint horizontal L73
  constraint vertical L74
  constraint horizontal L75
  constraint vertical L76
  constraint horizontal L77
  constraint vertical L78
  constraint perpendicular L69 L79
  constraint horizontal L80
  constraint vertical L81
  constraint horizontal L82
  constraint vertical L83
  constraint horizontal L84
  constraint vertical L85
  constraint horizontal L86
  constraint vertical L87
  constraint horizontal L88
  constraint vertical L89
  constraint horizontal L90
  constraint vertical L91
  constraint horizontal L92
  constraint vertical L93
  constraint horizontal L94
  constraint vertical L95
  constraint horizontal L96
  constraint vertical L97
  constraint horizontal L98
  constraint vertical L99
  constraint perpendicular L98 L100
  constraint horizontal L101
  constraint vertical L102
  constraint horizontal L103
  constraint vertical L104
  constraint vertical L117
  constraint horizontal L118
  constraint vertical L119
  constraint horizontal L120
  constraint horizontal L121
  constraint vertical L122
  constraint horizontal L123
  constraint vertical L124
  measures "d3" distance of P0 P1
  measures "d4" distance of P0 P2
  measures "d7" distance of P3 P4
  measures "d8" distance of P3 P5
  measures "d9" distance of L17.start P6
  measures "d10" distance of L17.start P7
  measures "d11" radius of A0
  measures "d14" diameter of A12
  measures "d18" diameter of A13
  measures "d21" diameter of A14
  measures "d24" diameter of A15
  measures "d32" distance of L12.start L12.end
  measures "d33" angle of L13 L14
  measures "d34" distance of L12.end L13.end
  measures "d35" distance of L12.end L15.end
  measures "d38" diameter of A16
  measures "d39" diameter of A17
  measures "d40" diameter of A18
  measures "d41" diameter of A19
  measures "d42" distance of L17.start L17.end
  measures "d43" distance of L17.end L18.end
  measures "d44" distance of L18.end P8
  measures "d45" distance of L18.end P9
  measures "d46" radius of A20
  measures "d47" radius of A21
  measures "d64" distance of L26.start L26.end
  measures "d107" distance of L35.end L37.end
  measures "d108" distance of L35.end L39.end
  measures "d109" distance of L37.end L41.end
  measures "d110" distance of L41.end L42.end
  measures "d111" distance of L41.end L44.end
  measures "d112" distance of L42.end L46.end
  measures "d113" distance of L46.end L47.end
  measures "d114" distance of L46.end L49.end
  measures "d115" distance of L39.end L51.end
  measures "d116" distance of L51.end L52.end
  measures "d117" distance of L51.end L54.end
  measures "d118" distance of L52.end L56.end
  measures "d119" distance of L56.end L57.end
  measures "d120" distance of L56.end L59.end
  measures "d121" distance of L57.end L61.end
  measures "d122" distance of L61.end L62.end
  measures "d123" distance of L61.end L64.end
  measures "d124" distance of L54.end L66.end
  measures "d125" distance of L66.end L67.end
  measures "d126" distance of L66.end L69.end
  measures "d127" distance of L71.start L71.end
  measures "d128" distance of L71.start L73.end
  measures "d129" distance of L75.start L75.end
  measures "d130" distance of L75.start L77.end
  measures "d131" distance of L69.end L79.end
  measures "d132" distance of L79.end L80.end
  measures "d133" distance of L79.end L82.end
  measures "d134" distance of L84.start L84.end
  measures "d135" distance of L84.start L86.end
  measures "d136" distance of L88.start L88.end
  measures "d137" distance of L88.start L90.end
  measures "d139" distance of L92.start L92.end
  measures "d140" distance of L92.start L94.end
  measures "d143" distance of L96.start L96.end
  measures "d144" distance of L96.start L98.end
  measures "d145" distance of L98.end L100.end
  measures "d146" distance of L100.end L101.end
  measures "d147" distance of L100.end L103.end
  measures "d175" diameter of A25
  measures "d186" distance of L96.end L120.end
extrude "Extrude11" add sketch "Sketch1" along normal blind 2 contours L0 L1 L2 L3 L6 A0 A3 A6 A9 L23 L25 L26 L27 L31 | L13 L15 L62 L63 L64 L65 | L35 L37 L38 L39 L40 | L42 L43 L44 L45 | L47 L48 L49 L50 | L52 L53 L54 L55 | L57 L58 L59 L60 | L67 L68 L69 L70 | L71 L72 L73 L74 | L75 L76 L77 L78 | L80 L81 L82 L83 | L84 L85 L86 L87 | L88 L89 L90 L91 | L92 L93 L94 L95 | L96 L97 L98 L99 | L101 L102 L103 L104 | S0 S1 S2 S3 S4 S5 S6 S7 S8 S9 S10 S11 L105 S12 S13 S14 S15 S16 S17 S18 S19 S20 S21 L106 S22 S23 S24 S25 S26 S27 S28 S29 S30 S31 S32 S33 S34 S35 L107 S36 S37 L108 S38 S39 S40 | S41 S42 S43 S44 S45 S46 S47 S48 S49 S50 S51 S52 S53 S54 S55 S56 S57 L109 S58 S59 S60 S61 S62 S63 S64 S65 S66 S67 S68 S69 S70 S71 | S72 S73 S74 S75 S76 S77 S78 S79 S80 S81 S82 S83 S84 S85 S86 S87 S88 L111 S89 S90 S91 S92 S93 S94 S95 S96 S97 S98 S99 S100 S101 S102 | S103 S104 A24 S105 S106 L113 | S107 S108 S109 S110 | S111 S112 S113 S114 | S115 S116 | S117 S118 | S119 S120 | S121 S122 | S123 S124 S125 S126 | S127 S128 S129 S130 | S131 S132 S133 S134 | S135 S136 S137 S138 | A25 | L117 L118 L119 L120 L121 L122 L123 L124 makes body 1
extrude "Extrude12" add sketch "Sketch1" along normal blind 2 contours L0 L1 L3 L4 L5 L6 L7 A0 A1 A3 A4 A6 A7 A9 A10 bodies 1
extrude "Extrude13" add sketch "Sketch1" along normal blind 4 contours L10 L21 L24 L28 L32 L33 | L8 L9 L10 L11 A2 A5 A8 A11 L19 L20 L21 L22 A20 A21 A22 A23 L30 L32 | A12 | A13 | A14 | A15 bodies 1 makes body 2 at (41, 0, 1.3333)
extrude "Extrude14" add sketch "Sketch1" along normal blind 5 contours L2 L6 L21 L26 L27 L30 L34 | L2 L6 L21 L23 L25 L26 L27 L28 L31 L34 | L10 L21 L29 L30 L34 | L10 L21 L24 L28 L29 L33 L34 bodies 1 2
extrude "Extrude15" add sketch "Sketch1" along normal blind 8 contours L10 L21 L24 L28 L32 L33 | L8 L9 L10 L11 A2 A5 A8 A11 L19 L20 L21 L22 A20 A21 A22 A23 L30 L32 bodies 1
extrude "Extrude16" add sketch "Sketch1" along normal blind 7 contours A16 | A17 | A18 | A19 bodies 1
extrude "Extrude17" add sketch "Sketch1" along normal blind 4 contours L12 L13 L64 | L12 L15 L64 | L13 L15 L16 L64 bodies 1
extrude "Extrude18" add sketch "Sketch1" along normal blind 9 contours L2 L4 L5 L6 L7 A1 A4 A7 A10 L19 L20 L21 L22 A20 A21 A22 A23 L30 L32 | L2 L6 L21 L23 L25 L28 L31 L32 bodies 1
extrude "Extrude19" add 1 faces at (88, 96.9667, 5) along direction (0, 0, 1) blind 1.5 on bodies 1 bodies 1
extrude "Extrude20" add 1 faces at (2.2058, 92.7538, 8) along direction (0, 0, 1) blind 1.5 on bodies 1 bodies 1
extrude "Extrude21" add 1 faces at (2.7058, 5.0462, 9) along direction (0, 0, 1) blind 1.5 on bodies 1 bodies 1
extrude "Extrude22" cut sketch "Sketch1" along normal blind 11 contours L2 L6 L21 L23 L25 L28 L31 L32 | L2 L6 L21 L23 L25 L26 L27 L28 L31 L34 | L10 L21 L24 L28 L32 L33 | L10 L21 L24 L28 L29 L33 L34 bodies 1
extrude "Extrude23" add sketch "Sketch1" along normal blind 6.5 contours L10 L21 L24 L28 L32 L33 | L10 L21 L24 L28 L29 L33 L34 bodies 1
extrude "Extrude24" add sketch "Sketch1" along normal blind 6.5 contours L2 L6 L21 L23 L25 L28 L31 L32 | L2 L6 L21 L23 L25 L26 L27 L28 L31 L34 bodies 1
extrude "Extrude25" add sketch "Sketch1" along normal blind 9.5 contours L10 L21 L29 L30 L34 bodies 1
extrude "Extrude26" add sketch "Sketch1" along normal blind 10.5 contours L2 L6 L21 L26 L27 L30 L34 bodies 1
extrude "Extrude27" add 1 faces at (2.7058, 5.0462, 10.5) along direction (0, 0, 1) blind 1 on bodies 1 bodies 1
extrude "Extrude28" add sketch "Sketch1" along normal blind 2 separate body contours L0 L1 L2 L3 L6 A0 A3 A6 A9 L23 L25 L26 L27 L31 | L0 L1 L3 L4 L5 L6 L7 A0 A1 A3 A4 A6 A7 A9 A10 | L2 L4 L5 L6 L7 A1 A4 A7 A10 L19 L20 L21 L22 A20 A21 A22 A23 L30 L32 | L2 L6 L21 L23 L25 L28 L31 L32 | L2 L6 L21 L26 L27 L30 L34 | L2 L6 L21 L23 L25 L26 L27 L28 L31 L34 | L10 L21 L24 L28 L32 L33 | L8 L9 L10 L11 A2 A5 A8 A11 L19 L20 L21 L22 A20 A21 A22 A23 L30 L32 | L10 L21 L29 L30 L34 | L10 L21 L24 L28 L29 L33 L34 | A12 | A13 | A14 | A15 | L12 L13 L64 | L12 L15 L64 | L13 L15 L16 L64 | L13 L15 L62 L63 L64 L65 | A16 | A17 | A18 | A19 | L35 L37 L38 L39 L40 | L42 L43 L44 L45 | L47 L48 L49 L50 | L52 L53 L54 L55 | L57 L58 L59 L60 | L67 L68 L69 L70 | L71 L72 L73 L74 | L75 L76 L77 L78 | L80 L81 L82 L83 | L84 L85 L86 L87 | L88 L89 L90 L91 | L92 L93 L94 L95 | L96 L97 L98 L99 | L101 L102 L103 L104 | S0 S1 S2 S3 S4 S5 S6 S7 S8 S9 S10 S11 L105 S12 S13 S14 S15 S16 S17 S18 S19 S20 S21 L106 S22 S23 S24 S25 S26 S27 S28 S29 S30 S31 S32 S33 S34 S35 L107 S36 S37 L108 S38 S39 S40 | S41 S42 S43 S44 S45 S46 S47 S48 S49 S50 S51 S52 S53 S54 S55 S56 S57 L109 S58 S59 S60 S61 S62 S63 S64 S65 S66 S67 S68 S69 S70 S71 | S72 S73 S74 S75 S76 S77 S78 S79 S80 S81 S82 S83 S84 S85 S86 S87 S88 L111 S89 S90 S91 S92 S93 S94 S95 S96 S97 S98 S99 S100 S101 S102 | S103 S104 A24 S105 S106 L113 | S107 S108 S109 S110 | S111 S112 S113 S114 | S115 S116 | S117 S118 | S119 S120 | S121 S122 | S123 S124 S125 S126 | S127 S128 S129 S130 | S131 S132 S133 S134 | S135 S136 S137 S138 | A25 | L117 L118 L119 L120 L121 L122 L123 L124 makes body 3
fillet "Fillet1" radius 2 8 edges at (56.5, 97.3, 2) (2.9289, 94.3711, 2) (0, 48.65, 2) (2.9289, 2.9289, 2) (56.5, 0, 2) (110.0711, 2.9289, 2) (113, 48.65, 2) (110.0711, 94.3711, 2) on bodies 3
move_body "Move1" bodies 3 to x (1, 0, 0) y (0, 1, 0) z (0, 0, 1) at (0, 0, 2)
extrude "Extrude29" add sketch "Sketch1" along normal blind 2 contours L10 L21 L24 L28 L32 L33 | L8 L9 L10 L11 A2 A5 A8 A11 L19 L20 L21 L22 A20 A21 A22 A23 L30 L32 | L10 L21 L29 L30 L34 | L10 L21 L24 L28 L29 L33 L34 bodies 3
move_body "Move2" bodies 3 to x (1, 0, 0) y (0, 1, 0) z (0, 0, 1) at (0, 0, 9.5)
extrude "Extrude30" cut sketch "Sketch1" along normal blind 16 contours L12 L13 L64 | L12 L15 L64 | L13 L15 L62 L63 L64 L65 | L35 L37 L38 L39 L40 | L42 L43 L44 L45 | L47 L48 L49 L50 | L52 L53 L54 L55 | L57 L58 L59 L60 | L67 L68 L69 L70 | L71 L72 L73 L74 | L75 L76 L77 L78 | L80 L81 L82 L83 | L84 L85 L86 L87 | L88 L89 L90 L91 | L92 L93 L94 L95 | L96 L97 L98 L99 | L101 L102 L103 L104 | S41 S42 S43 S44 S45 S46 S47 S48 S49 S50 S51 S52 S53 S54 S55 S56 S57 L109 S58 S59 S60 S61 S62 S63 S64 S65 S66 S67 S68 S69 S70 S71 | S72 S73 S74 S75 S76 S77 S78 S79 S80 S81 S82 S83 S84 S85 S86 S87 S88 L111 S89 S90 S91 S92 S93 S94 S95 S96 S97 S98 S99 S100 S101 S102 | S103 S104 A24 S105 S106 L113 | S107 S108 S109 S110 | S111 S112 S113 S114 | S115 S116 | S117 S118 | S119 S120 | S121 S122 | S123 S124 S125 S126 | S127 S128 S129 S130 | S131 S132 S133 S134 | S135 S136 S137 S138 bodies 3
move_body "Move3" bodies 3 to x (1, 0, 0) y (0, 1, 0) z (0, 0, 1) at (0, 0, -9.5)
extrude "Extrude31" cut sketch "Sketch1" along normal blind 2 contours L2 L6 L21 L23 L25 L28 L31 L32 | L2 L6 L21 L23 L25 L26 L27 L28 L31 L34 | L10 L21 L24 L28 L32 L33 | L10 L21 L24 L28 L29 L33 L34 bodies 3
extrude "Extrude32" add 1 faces at (84, 96.6333, 6.5) along direction (0, 0, 1) blind 2 on bodies 1 bodies 1
extrude "Extrude33" cut 1 faces at (84, 96.6333, 8.5) along direction (0, 0, -1) blind 0.5 on bodies 1 bodies 1
extrude "Extrude34" cut 1 faces at (2.2058, 92.7538, 9.5) along direction (0, 0, -1) blind 9.5 on bodies 1 bodies 1
extrude "Extrude35" cut 1 faces at (2.7058, 5.0462, 11.5) along direction (0, 0, -1) blind 11.5 on bodies 1 bodies 1
extrude "Extrude36" cut 1 faces at (84, 96.6333, 8) along direction (0, 0, -1) blind 9 on bodies 1 bodies 1
extrude "Extrude37" add sketch "Sketch1" along normal blind 8.6 contours L2 L4 L5 L6 L7 A1 A4 A7 A10 L19 L20 L21 L22 A20 A21 A22 A23 L30 L32 bodies 1
extrude "Extrude38" add sketch "Sketch1" along normal blind 6.6 contours L8 L9 L10 L11 A2 A5 A8 A11 L19 L20 L21 L22 A20 A21 A22 A23 L30 L32 bodies 1
extrude "Extrude39" add sketch "Sketch1" along normal blind 8.6 contours L2 L6 L21 L26 L27 L30 L34 bodies 1
extrude "Extrude40" add sketch "Sketch1" along normal blind 6.6 contours L10 L21 L29 L30 L34 bodies 1
extrude "Extrude41" add sketch "Sketch1" along normal blind 5.1 contours L2 L6 L21 L23 L25 L28 L31 L32 | L2 L6 L21 L23 L25 L26 L27 L28 L31 L34 | L10 L21 L24 L28 L32 L33 | L10 L21 L24 L28 L29 L33 L34 bodies 1
move_body "Move4" bodies 3 to x (1, 0, 0) y (0, 1, 0) z (0, 0, 1) at (0, 0, 6.6)
extrude "Extrude42" cut 4 faces at (7.0311, 82.0151, 7) (7.3443, 13.9653, 7) (104.6557, 82.1411, 7) (105.412, 13.2953, 7) along direction (0, 0, -1) blind 3 on bodies 1 bodies 1
extrude "Extrude43" add sketch "Sketch1" along normal blind 8.6 contours A25 bodies 3
extrude "Extrude44" cut 1 faces at (100.4276, 85.6907, 0) along direction (0, 0, 1) blind 5.6 on bodies 3 bodies 3
extrude "Extrude45" add 1 faces at (84, 96.6333, 5.1) along direction (0, 0, 1) blind 0.5 on bodies 1 bodies 1
extrude "Extrude48" add sketch "Sketch1" along normal blind 8.6 contours L117 L118 L119 L120 L121 L122 L123 L124 bodies 3
extrude "Extrude49" cut sketch "Sketch1" along normal blind 5.6 contours L117 L118 L119 L120 L121 L122 L123 L124 bodies 3
extrude "Extrude50" add 1 faces at (2.7058, 5.0462, 8.6) along direction (0, 0, 1) blind 2 on bodies 1 bodies 1
extrude "Extrude51" add 1 faces at (2.2058, 92.7538, 6.6) along direction (0, 0, 1) blind 2 on bodies 1 bodies 1
extrude "Extrude52" add 1 faces at (84, 96.6333, 5.6) along direction (0, 0, 1) blind 2 on bodies 1 bodies 1
extrude "Extrude53" cut 1 faces at (84, 96.6333, 7.6) along direction (0, 0, -1) blind 1 on bodies 1 bodies 1
named bodies: "Case", "Lid"
